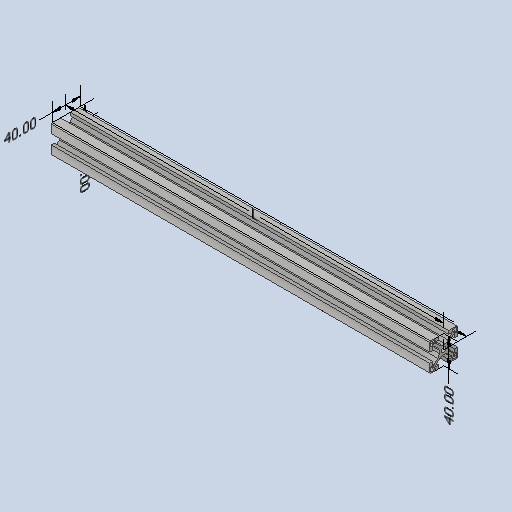
# Autodesk Inventor part: Robotunits Profil 40 x 40 - PIL 4040 SNN 0540
Saved by Autodesk Inventor 2023 (Build 270158000, 158)
## iProperties
Created: 2023-08-22
Part Number: Robotunits Profil 40 x 40 - PIL 4040 SNN 0540
Material: Generic
Catalog Web Link: www.cadenas.de
Description: PIL 4040-Extrusion 40 x 40
Vendor: ROBOTUNITS
Document SubType Name: Modeling
Designer: psAdmin
Manufacturer: ROBOTUNITS
Mass: 826.2 g
Surface Area: 2256.05 cm^2
Volume: 304.452 cm^3
Density: 2.7 g/cm^3
Appearance: PSOLRGB-175-175-175
Category: PARTsolutions
Company: ROBOTUNITS
PSOL_IDENT_0: {$CADENAS_DATA/23d-libs/robotunits/pool_bauteile/pil_4040.prj},234 {VTYP=3D},{NB=Robotunits Profil 4
PSOL_IDENT_1: 0 x 40 - PIL 4040 SNN 0540},{LINA=Robotunits Profil 40 x 40 - PIL 4040 SNN 0540},{NN=PIL 4040},{DATE=
PSOL_IDENT_2: 21.08.2023 10:38:56},{GEOMDATE=21.08.2023 10:38:50},{VERSION=},{LINEID=10},{WBVAR=L},{WBNUMERIC=L}
PSOL_IDENT_3: {NB=Robotunits Profil 40 x 40 - PIL 4040 SNN 0540},{LINA=Robotunits Profil 40 x 40 - PIL 4040 SNN 05
PSOL_IDENT_4: 40},{KT=DUMMY},{ARTIKEL=Profil 40 x 40},{L=540.0},{LMAX=6000},{GEW=0.826},{LX=0540},{LXX=100,[40:600
PSOL_IDENT_5: 0]},{ROB=PIL4040},{ROBX=http://www.robotunits.com/$CADENAS_LANGUAGE./Webshop/Profiltechnik/shopitem/
PSOL_IDENT_6: profilstange-40x40-laenge-bis-6050-mm/90/},{ZOLL=76042990}
NB: Robotunits Profil 40 x 40 - PIL 4040 SNN 0540
NN: PIL 4040
NT: Extrusion 40 x 40
NBSYN: Robotunits $ARTIKEL. - PIL 4040 SNN $LX.
LINA: Robotunits Profil 40 x 40 - PIL 4040 SNN 0540
CATALOG: Robotunits
ARTIKEL: Extrusion 40 x 40
L: 540
LMAX: 6000
GEW: 0.826
ROB: PIL4040
ZOLL: 76042990
SUPPLIER: ROBOTUNITS
ARTICLENO: Robotunits Profil 40 x 40 - PIL 4040 SNN 0540
BOMINFO: Robotunits Profil 40 x 40 - PIL 4040 SNN 0540
CREATOR: CADENAS GmbH
Title: Robotunits Profil 40 x 40 - PIL 4040 SNN 0540
Author: Cadenas PARTsolutions
Comments: Extrusion 40 x 40
Autodesk Inventor part; units mm, degrees
sketch "Skizze_1" plane through (0, 0, 0) normal (1, 0, 0) x (0, 1, 0)
  line L0 (18.75, 20) -> (7, 20)
  line L1 (7, 20) -> (7, 15.5)
  line L2 (7, 15.5) -> (11.7, 15.5)
  line L3 (11.7, 15.5) -> (11.7, 13.82)
  line L4 (11.7, 13.82) -> (6.4481, 8.5681)
  line L5 (6.4481, 8.5681) -> (2, 6)
  line L6 (2, 6) -> (-2, 6)
  line L7 (-2, 6) -> (-6.4481, 8.5681)
  line L8 (-6.4481, 8.5681) -> (-11.7, 13.82)
  line L9 (-11.7, 13.82) -> (-11.7, 15.5)
  line L10 (-11.7, 15.5) -> (-7, 15.5)
  line L11 (-7, 15.5) -> (-7, 20)
  line L12 (-7, 20) -> (-18.75, 20)
  line L13 (-18.75, 20) -> (-20, 18.75)
  line L14 (-20, 18.75) -> (-20, 7)
  line L15 (-20, 7) -> (-15.5, 7)
  line L16 (-15.5, 7) -> (-15.5, 11.7)
  line L17 (-15.5, 11.7) -> (-13.82, 11.7)
  line L18 (-13.82, 11.7) -> (-8.5681, 6.4481)
  line L19 (-8.5681, 6.4481) -> (-6, 2)
  line L20 (-6, 2) -> (-6, -2)
  line L21 (-6, -2) -> (-8.5681, -6.4481)
  line L22 (-8.5681, -6.4481) -> (-13.82, -11.7)
  line L23 (-13.82, -11.7) -> (-15.5, -11.7)
  line L24 (-15.5, -11.7) -> (-15.5, -7)
  line L25 (-15.5, -7) -> (-20, -7)
  line L26 (-20, -7) -> (-20, -18.75)
  line L27 (-20, -18.75) -> (-18.75, -20)
  line L28 (-18.75, -20) -> (-7, -20)
  line L29 (-7, -20) -> (-7, -15.5)
  line L30 (-7, -15.5) -> (-11.7, -15.5)
  line L31 (-11.7, -15.5) -> (-11.7, -13.82)
  line L32 (-11.7, -13.82) -> (-6.4481, -8.5681)
  line L33 (-6.4481, -8.5681) -> (-2, -6)
  line L34 (-2, -6) -> (2, -6)
  line L35 (2, -6) -> (6.4481, -8.5681)
  line L36 (6.4481, -8.5681) -> (11.7, -13.82)
  line L37 (11.7, -13.82) -> (11.7, -15.5)
  line L38 (11.7, -15.5) -> (7, -15.5)
  line L39 (7, -15.5) -> (7, -20)
  line L40 (7, -20) -> (18.75, -20)
  line L41 (18.75, -20) -> (20, -18.75)
  line L42 (20, -18.75) -> (20, -7)
  line L43 (20, -7) -> (15.5, -7)
  line L44 (15.5, -7) -> (15.5, -11.7)
  line L45 (15.5, -11.7) -> (13.82, -11.7)
  line L46 (13.82, -11.7) -> (8.5681, -6.4481)
  line L47 (8.5681, -6.4481) -> (6, -2)
  line L48 (6, -2) -> (6, 2)
  line L49 (6, 2) -> (8.5681, 6.4481)
  line L50 (8.5681, 6.4481) -> (13.82, 11.7)
  line L51 (13.82, 11.7) -> (15.5, 11.7)
  line L52 (15.5, 11.7) -> (15.5, 7)
  line L53 (15.5, 7) -> (20, 7)
  line L54 (20, 7) -> (20, 18.75)
  line L55 (20, 18.75) -> (18.75, 20)
  line L56 (17.75, -12.1) -> (17.1, -12.1)
  line L57 (17.1, -12.1) -> (15.45, -13.75)
  line L58 (15.45, -13.75) -> (14.5, -13.75)
  arc A0 (14.5, -13.75) -> (13.75, -14.5) centre (14.5, -14.5) ccw
  line L59 (13.75, -14.5) -> (13.75, -15.45)
  line L60 (13.75, -15.45) -> (12.1, -17.1)
  line L61 (12.1, -17.1) -> (12.1, -17.75)
  arc A1 (12.1, -17.75) -> (12.85, -18.5) centre (12.85, -17.75) ccw
  line L62 (12.85, -18.5) -> (17.5, -18.5)
  arc A2 (17.5, -18.5) -> (18.5, -17.5) centre (17.5, -17.5) ccw
  line L63 (18.5, -17.5) -> (18.5, -12.85)
  arc A3 (18.5, -12.85) -> (17.75, -12.1) centre (17.75, -12.85) ccw
  line L64 (-17.1, -12.1) -> (-17.75, -12.1)
  arc A4 (-17.75, -12.1) -> (-18.5, -12.85) centre (-17.75, -12.85) ccw
  line L65 (-18.5, -12.85) -> (-18.5, -17.5)
  arc A5 (-18.5, -17.5) -> (-17.5, -18.5) centre (-17.5, -17.5) ccw
  line L66 (-17.5, -18.5) -> (-12.85, -18.5)
  arc A6 (-12.85, -18.5) -> (-12.1, -17.75) centre (-12.85, -17.75) ccw
  line L67 (-12.1, -17.75) -> (-12.1, -17.1)
  line L68 (-12.1, -17.1) -> (-13.75, -15.45)
  line L69 (-13.75, -15.45) -> (-13.75, -14.5)
  arc A7 (-13.75, -14.5) -> (-14.5, -13.75) centre (-14.5, -14.5) ccw
  line L70 (-14.5, -13.75) -> (-15.45, -13.75)
  line L71 (-15.45, -13.75) -> (-17.1, -12.1)
  circle A8 centre (0, 0) radius 3.5
  arc A9 (-17.5, 18.5) -> (-18.5, 17.5) centre (-17.5, 17.5) ccw
  line L72 (-18.5, 17.5) -> (-18.5, 12.85)
  arc A10 (-18.5, 12.85) -> (-17.75, 12.1) centre (-17.75, 12.85) ccw
  line L73 (-17.75, 12.1) -> (-17.1, 12.1)
  line L74 (-17.1, 12.1) -> (-15.45, 13.75)
  line L75 (-15.45, 13.75) -> (-14.5, 13.75)
  arc A11 (-14.5, 13.75) -> (-13.75, 14.5) centre (-14.5, 14.5) ccw
  line L76 (-13.75, 14.5) -> (-13.75, 15.45)
  line L77 (-13.75, 15.45) -> (-12.1, 17.1)
  line L78 (-12.1, 17.1) -> (-12.1, 17.75)
  arc A12 (-12.1, 17.75) -> (-12.85, 18.5) centre (-12.85, 17.75) ccw
  line L79 (-12.85, 18.5) -> (-17.5, 18.5)
  line L80 (17.5, 18.5) -> (12.85, 18.5)
  arc A13 (12.85, 18.5) -> (12.1, 17.75) centre (12.85, 17.75) ccw
  line L81 (12.1, 17.75) -> (12.1, 17.1)
  line L82 (12.1, 17.1) -> (13.75, 15.45)
  line L83 (13.75, 15.45) -> (13.75, 14.5)
  arc A14 (13.75, 14.5) -> (14.5, 13.75) centre (14.5, 14.5) ccw
  line L84 (14.5, 13.75) -> (15.45, 13.75)
  line L85 (15.45, 13.75) -> (17.1, 12.1)
  line L86 (17.1, 12.1) -> (17.75, 12.1)
  arc A15 (17.75, 12.1) -> (18.5, 12.85) centre (17.75, 12.85) ccw
  line L87 (18.5, 12.85) -> (18.5, 17.5)
  arc A16 (18.5, 17.5) -> (17.5, 18.5) centre (17.5, 17.5) ccw
  constraints: 176 end point, 32 point on circle, 17 centre point
extrude "Extrusion1" add sketch "Skizze_1" along normal blind 540
ref_plane "CS_ANBAU_HINTEN_LINKS_XY" through (540, 0, 20) normal (1, 0, 0) x (0, 0, -1)
ref_plane "CS_ANBAU_HINTEN_LINKS_YZ" through (540, 0, 20) normal (0, 0, -1) x (0, 1, 0)
ref_plane "CS_ANBAU_HINTEN_LINKS_ZX" through (540, 0, 20) normal (0, 1, 0) x (1, 0, 0)
ref_plane "CS_ANBAU_HINTEN_OBEN_XY" through (540, 20, 0) normal (1, 0, 0) x (0, 0, -1)
ref_plane "CS_ANBAU_HINTEN_OBEN_YZ" through (540, 20, 0) normal (0, 0, -1) x (0, 1, 0)
ref_plane "CS_ANBAU_HINTEN_OBEN_ZX" through (540, 20, 0) normal (0, 1, 0) x (1, 0, 0)
ref_plane "CS_ANBAU_HINTEN_RECHTS_XY" through (540, 0, -20) normal (1, 0, 0) x (0, 0, -1)
ref_plane "CS_ANBAU_HINTEN_RECHTS_YZ" through (540, 0, -20) normal (0, 0, -1) x (0, 1, 0)
ref_plane "CS_ANBAU_HINTEN_RECHTS_ZX" through (540, 0, -20) normal (0, 1, 0) x (1, 0, 0)
ref_plane "CS_ANBAU_HINTEN_UNTEN_XY" through (540, -20, 0) normal (1, 0, 0) x (0, 0, -1)
ref_plane "CS_ANBAU_HINTEN_UNTEN_YZ" through (540, -20, 0) normal (0, 0, -1) x (0, 1, 0)
ref_plane "CS_ANBAU_HINTEN_UNTEN_ZX" through (540, -20, 0) normal (0, 1, 0) x (1, 0, 0)
ref_plane "CS_ANBAU_QUER_XY" through (0, 0, 20) normal (0, 0, 1) x (1, 0, 0)
ref_plane "CS_ANBAU_QUER_YZ" through (0, 0, 20) normal (1, 0, 0) x (0, 1, 0)
ref_plane "CS_ANBAU_QUER_ZX" through (0, 0, 20) normal (0, 1, 0) x (0, 0, 1)
ref_plane "CS_ANBAU_QUER_1_XY" through (540, 0, 20) normal (0, 0, 1) x (1, 0, 0)
ref_plane "CS_ANBAU_QUER_1_YZ" through (540, 0, 20) normal (1, 0, 0) x (0, 1, 0)
ref_plane "CS_ANBAU_QUER_1_ZX" through (540, 0, 20) normal (0, 1, 0) x (0, 0, 1)
ref_plane "CS_ANBAU_VORNE_LINKS_XY" through (0, 0, 20) normal (-1, 0, 0) x (0, 0, -1)
ref_plane "CS_ANBAU_VORNE_LINKS_YZ" through (0, 0, 20) normal (0, 0, -1) x (0, -1, 0)
ref_plane "CS_ANBAU_VORNE_LINKS_ZX" through (0, 0, 20) normal (0, -1, 0) x (-1, 0, 0)
ref_plane "CS_ANBAU_VORNE_OBEN_XY" through (0, 20, 0) normal (-1, 0, 0) x (0, 0, -1)
ref_plane "CS_ANBAU_VORNE_OBEN_YZ" through (0, 20, 0) normal (0, 0, -1) x (0, -1, 0)
ref_plane "CS_ANBAU_VORNE_OBEN_ZX" through (0, 20, 0) normal (0, -1, 0) x (-1, 0, 0)
ref_plane "CS_ANBAU_VORNE_RECHTS_XY" through (0, 0, -20) normal (-1, 0, 0) x (0, 0, -1)
ref_plane "CS_ANBAU_VORNE_RECHTS_YZ" through (0, 0, -20) normal (0, 0, -1) x (0, -1, 0)
ref_plane "CS_ANBAU_VORNE_RECHTS_ZX" through (0, 0, -20) normal (0, -1, 0) x (-1, 0, 0)
ref_plane "CS_ANBAU_VORNE_UNTEN_XY" through (0, -20, 0) normal (-1, 0, 0) x (0, 0, -1)
ref_plane "CS_ANBAU_VORNE_UNTEN_YZ" through (0, -20, 0) normal (0, 0, -1) x (0, -1, 0)
ref_plane "CS_ANBAU_VORNE_UNTEN_ZX" through (0, -20, 0) normal (0, -1, 0) x (-1, 0, 0)
ref_plane "p1_XY" through (0, 20, 0) normal (0, 0, 1) x (1, 0, 0)
ref_plane "p1_YZ" through (0, 20, 0) normal (1, 0, 0) x (0, 1, 0)
ref_plane "p1_ZX" through (0, 20, 0) normal (0, 1, 0) x (0, 0, 1)
ref_plane "p2_XY" through (540, 20, 0) normal (0, 0, 1) x (1, 0, 0)
ref_plane "p2_YZ" through (540, 20, 0) normal (1, 0, 0) x (0, 1, 0)
ref_plane "p2_ZX" through (540, 20, 0) normal (0, 1, 0) x (0, 0, 1)
ref_plane "p3_XY" through (540, -20, 18.75) normal (1, 0, 0) x (0, 0, -1)
ref_plane "p3_YZ" through (540, -20, 18.75) normal (0, 0, -1) x (0, 1, 0)
ref_plane "p3_ZX" through (540, -20, 18.75) normal (0, 1, 0) x (1, 0, 0)
ref_plane "p4_XY" through (540, 20, 18.75) normal (1, 0, 0) x (0, 0, -1)
ref_plane "p4_YZ" through (540, 20, 18.75) normal (0, 0, -1) x (0, 1, 0)
ref_plane "p4_ZX" through (540, 20, 18.75) normal (0, 1, 0) x (1, 0, 0)
ref_plane "p5_XY" through (540, 20, -21.25) normal (1, 0, 0) x (0, 0, -1)
ref_plane "p5_YZ" through (540, 20, -21.25) normal (0, 0, -1) x (0, 1, 0)
ref_plane "p5_ZX" through (540, 20, -21.25) normal (0, 1, 0) x (1, 0, 0)
ref_plane "pm1_XY" through (0, 0, 0) normal (1, 0, 0) x (0, 0, -1)
ref_plane "pm1_YZ" through (0, 0, 0) normal (0, 0, -1) x (0, 1, 0)
ref_plane "pm1_ZX" through (0, 0, 0) normal (0, 1, 0) x (1, 0, 0)
ref_plane "pm2_XY" through (540, 0, -1.25) normal (1, 0, 0) x (0, 0, -1)
ref_plane "pm2_YZ" through (540, 0, -1.25) normal (0, 0, -1) x (0, 1, 0)
ref_plane "pm2_ZX" through (540, 0, -1.25) normal (0, 1, 0) x (1, 0, 0)
body "Solid1"
